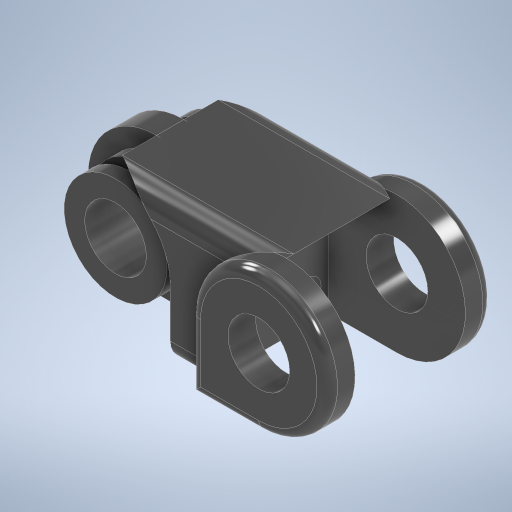
# Autodesk Inventor part: MiddlePart
Saved by Autodesk Inventor 2024 (Build 280153000, 153)
## iProperties
Created: 2024-03-20
Part Number: MiddlePart
Material: Generic
Document SubType Name: Modeling
Designer: Wojtek
Density: 1 g/cm^3
Appearance: Default
Author: Wojtek
Autodesk Inventor part; units mm, degrees
ref_plane "YZ Plane" through (0, 0, 0) normal (1, 0, 0) x (0, 1, 0)
ref_plane "XZ Plane" through (0, 0, 0) normal (0, 1, 0) x (-1, 0, 0)
ref_plane "XY Plane" through (0, 0, 0) normal (0, 0, 1) x (1, 0, 0)
sketch "Sketch1" plane through (0, 0, 0) normal (0, 0, 1) x (1, 0, 0)
  circle A0 centre (0, 0) radius 10
  line L0 (0, 10) -> (25, 10)
  circle A1 centre (25, 0) radius 10
  line L1 (0, -10) -> (25, -10)
  line L2 (10, 0) -> (10, -10)
  line L3 (15, 0) -> (15, -10)
  circle A2 centre (0, 0) radius 3.5
  circle A3 centre (25, 0) radius 3.5
  circle A4 centre (0, 0) radius 7.5
  circle A5 centre (0, 0) radius 6
  circle A6 centre (0, 0) radius 4.5
  circle A7 centre (25, 0) radius 4.5
  dimension "d0" = 20
  dimension "d1" = 25
  dimension "d2" = 20
  dimension "d3" = 25
  dimension "d4" = 10
  dimension "d5" = 7
  dimension "d6" = 7
  dimension "d7" = 15
  dimension "d8" = 12
  dimension "d33" = 9
  dimension "d34" = 9
  constraints: 8 centre point, 8 end point, 7 coincident, 6 point on circle, 4 tangent, 2 point on line, 1 horizontal, 1 perpendicular, 1 vertical
  measures "d0" diameter of A0
  measures "d1" distance of L0.start L0.end
  measures "d2" diameter of A1
  measures "d3" distance of L1.start L1.end
  measures "d4" distance from line of point (0, 0) L1
  measures "d5" diameter of A2
  measures "d6" diameter of A3
  measures "d7" diameter of A4
  measures "d8" diameter of A5
  measures "d33" diameter of A6
  measures "d34" diameter of A7
extrude "Extrusion1" add sketch "Sketch1" along normal mid plane 20 contours A0 L0 A1 L3 L1 L2
extrude "Extrusion2" add sketch "Sketch1" along normal mid plane 4 contours A0 | A4 | A5 | A6
extrude "Extrusion3" add sketch "Sketch1" along normal mid plane 8 contours A4 | A5 | A6
extrude "Extrusion4" add sketch "Sketch1" along normal mid plane 12 contours A5 | A6
sketch "Sketch2" plane through (0, 0, 6) normal (0, 0, 1) x (1, 0, 0)
  circle A0 centre (0, 0) radius 7.5
  circle A1 centre (0, 0) radius 3.5
  dimension "d17" = 15
  dimension "d19" = 7
  constraints: 2 centre point, 2 coincident
  measures "d17" diameter of A0
  measures "d19" diameter of A1
sketch "Sketch3" plane through (0, 0, -6) normal (0, 0, -1) x (-1, 0, 0)
  circle A0 centre (0, 0) radius 7.5
  circle A1 centre (0, 0) radius 3.5
  dimension "d18" = 15
  dimension "d20" = 7
  constraints: 2 centre point, 2 coincident
  measures "d18" diameter of A0
  measures "d20" diameter of A1
extrude "Extrusion5" add sketch "Sketch3" along normal blind 2
extrude "Extrusion6" add sketch "Sketch2" along normal blind 2
extrude "Extrusion7" add sketch "Sketch1" along normal mid plane 4 contours L2 L1 A0
extrude "Extrusion8" add sketch "Sketch1" along normal mid plane 22 contours A1 | L3 A1 L1 | A7
extrude "Extrusion9" cut sketch "Sketch1" along normal mid plane 16.1 contours A1 | L3 A1 L1 | A7
fillet "Fillet1" radius 3 4 edges at (12.5, 10, 10) (12.5, 10, -10) (12.5, -10, 10) (12.5, -10, -10)
fillet "Fillet2" radius 1 6 edges at (32.0711, 7.0711, 11) (20, -10, 11) (15, -5, 11) (20, -10, -11) (15, -5, -11) (32.0711, 7.0711, -11)
extrude "Extrusion10" cut sketch "Sketch1" along normal mid plane 25 contours A2 | A3 | A6 | A7
extrude "Extrusion11" add sketch "Sketch1" along normal mid plane 24.2 contours A1 | L3 A1 L1
extrude "Extrusion12" cut sketch "Sketch1" along normal mid plane 16.1 contours A1 | L3 A1 L1
fillet "Fillet3" radius 1.5 6 edges at (15, -5, 12.1) (20, -10, 12.1) (32.0711, 7.0711, 12.1) (20, -10, -12.1) (15, -5, -12.1) (32.0711, 7.0711, -12.1)
sketch "Sketch4" plane through (15, -9.8102, -8.05) normal (1, 0, 0) x (0, 0, -1)
  line L0 (-16.1, 9.8102) -> (0, 9.8102) projected
  line L1 (-8.05, 9.8102) -> (-8.05, 12.3416) construction
  point P0 (-13.05, 9.8102)
  point P1 (-3.05, 9.8102)
  point P2 (-13.05, 15.81)
  point P3 (-3.05, 15.81)
  point P4 (-13.05, 3.81)
  point P5 (-3.05, 3.81)
  dimension "d42" = 5
  dimension "d43" = 2.5314
  dimension "d44" = 5.9997
  dimension "d59" = 6.0003
  dimension "d60" = 5
  constraints: 3 midpoint, 3 symmetric about line, 2 end point, 1 point on line, 1 vertical
  measures "d42" distance of point (-8.05, 9.81) point (-13.05, 9.81)
  measures "d43" vertical distance of point (-13.05, 9.81) L1.end
  measures "d44" distance of point (-13.05, 9.81) point (-13.05, 15.81)
  measures "d59" vertical distance of point (-8.05, 9.81) point (-13.05, 3.81)
  measures "d60" horizontal distance of point (-13.05, 3.81) point (-8.05, 9.81)
hole "Hole1" at (15, 5.9998, 5) at (15, 5.9998, -5) direction (-1, 0, 0) diameter 2 depth 8 tip angle 118
hole "Hole2" at (15, 5.9998, 5) at (15, 5.9998, -5) direction (1, 0, 0) diameter 2 depth 8 tip angle 118
hole "Hole3" at (15, -6.0002, 5) at (15, -6.0002, -5) direction (-1, 0, 0) diameter 2 depth 6 tip angle 118
fillet "Fillet4" radius 1 8 edges at (17.0482, 6.0638, 4.0021) (17.0482, 6.0638, -5.9979) (15, -6.0002, 6) (15, -6.0002, -4) (10, -6.0002, -4) (7.9523, 6.0631, -4.002) (7.9523, 6.0631, 5.998) (10, -6.0002, 6)
body "Solid1"
